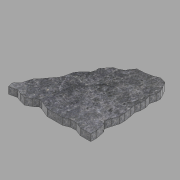
# Autodesk Inventor part: 1xRNDxRND-1074sqft
Saved by Autodesk Inventor 2022.2 (Build 262287000, 287)
## iProperties
Created: 2022-02-10
Part Number: 1xRNDxRND-1074sqft
Material: Granite, Cut, Polished
Document SubType Name: Modeling
Designer: awelt
Density: 2.7 g/cm^3
Appearance: Kasota SN sapphire
Author: awelt
Autodesk Inventor part; units mm, degrees
ref_plane "YZ Plane" through (0, 0, 0) normal (1, 0, 0) x (0, 1, 0)
ref_plane "XZ Plane" through (0, 0, 0) normal (0, 1, 0) x (-1, 0, 0)
ref_plane "XY Plane" through (0, 0, 0) normal (0, 0, 1) x (1, 0, 0)
sketch "Sketch2" plane through (0, 0, 0) normal (0, 1, 0) x (-1, 0, 0)
  line L0 (149.9475, 163.8702) -> (122.1528, 157.4561)
  line L1 (122.1528, 157.4561) -> (107.1865, 163.8702)
  line L2 (107.1865, 163.8702) -> (84.7369, 169.2153)
  line L3 (84.7369, 169.2153) -> (64.4255, 158.5251)
  line L4 (64.4255, 158.5251) -> (51.5972, 147.8348)
  line L5 (51.5972, 147.8348) -> (39.8379, 149.9729)
  line L6 (39.8379, 149.9729) -> (6.6981, 163.8702)
  line L7 (6.6981, 163.8702) -> (-30.7177, 163.8702)
  line L8 (-30.7177, 163.8702) -> (-49.9602, 163.8702)
  line L9 (-49.9602, 163.8702) -> (-71.3407, 155.318)
  line L10 (-71.3407, 155.318) -> (-91.6521, 154.249)
  line L11 (-91.6521, 154.249) -> (-117.3087, 163.8702)
  line L12 (-117.3087, 163.8702) -> (-140.8273, 163.8702)
  line L13 (-140.8273, 163.8702) -> (-155.7936, 163.8702)
  line L14 (-155.7936, 163.8702) -> (-155.7936, 141.4207)
  line L15 (-155.7936, 141.4207) -> (-149.3795, 109.35)
  line L16 (-149.3795, 109.35) -> (-139.7583, 97.5907)
  line L17 (-139.7583, 97.5907) -> (-145.1034, 77.2792)
  line L18 (-145.1034, 77.2792) -> (-152.5866, 52.6916)
  line L19 (-152.5866, 52.6916) -> (-152.5866, 34.5182)
  line L20 (-152.5866, 34.5182) -> (-148.3105, 7.7926)
  line L21 (-148.3105, 7.7926) -> (-144.0344, -11.4498)
  line L22 (-144.0344, -11.4498) -> (-148.3105, -27.4852)
  line L23 (-148.3105, -48.8657) -> (-141.8963, -68.1081)
  line L24 (-141.8963, -68.1081) -> (-148.3105, -89.4886)
  line L25 (-148.3105, -89.4886) -> (-148.3105, -103.386)
  line L26 (-148.3105, -103.386) -> (-138.6892, -121.5594)
  line L27 (-138.6892, -121.5594) -> (-127.999, -139.7328)
  line L28 (-127.999, -139.7328) -> (-106.6185, -146.147)
  line L29 (-106.6185, -146.147) -> (-84.169, -137.5948)
  line L30 (-84.169, -137.5948) -> (-58.5124, -132.2496)
  line L31 (-58.5124, -132.2496) -> (-32.8558, -131.1806)
  line L32 (-32.8558, -131.1806) -> (-18.9585, -111.9382)
  line L33 (-18.9585, -111.9382) -> (-15.7514, -104.455)
  line L34 (-15.7514, -104.455) -> (2.422, -94.8338)
  line L35 (2.422, -94.8338) -> (15.2503, -91.6267)
  line L36 (15.2503, -91.6267) -> (39.8379, -61.694)
  line L37 (39.8379, -61.694) -> (38.7689, -48.8657)
  line L38 (38.7689, -48.8657) -> (43.045, -34.9684)
  line L39 (43.045, -34.9684) -> (62.2874, -17.864)
  line L40 (62.2874, -17.864) -> (74.0467, -0.7596)
  line L41 (74.0467, -0.7596) -> (79.7125, 27.142)
  line L42 (79.7125, 27.142) -> (84.7369, 39.8633)
  line L43 (84.7369, 39.8633) -> (99.7033, 59.1058)
  line L44 (99.7033, 59.1058) -> (117.8767, 83.6934)
  line L45 (117.8767, 83.6934) -> (128.567, 95.4526)
  line L46 (128.567, 95.4526) -> (132.8431, 110.419)
  line L47 (132.8431, 110.419) -> (138.1882, 130.7305)
  line L48 (138.1882, 130.7305) -> (149.9475, 140.3517)
  line L49 (149.9475, 140.3517) -> (154.2236, 147.8348)
  line L50 (-148.3105, -27.4852) -> (-148.3105, -48.8657)
  line L51 (154.2236, 147.8348) -> (149.9475, 163.8702)
  point P0 (0, 0)
  constraints: 104 end point, 1 point on line, 1 vertical
extrude "Extrusion1" add sketch "Sketch2" along normal blind 25.4
body "Solid1"
